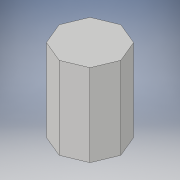
# Autodesk Inventor part: pin_4mm
Saved by Autodesk Inventor 2019 (Build 230136000, 136)
## iProperties
Created: 2019-05-07
Part Number: pin_4mm
Material: Generic
Document SubType Name: Modeling
Designer: assman
Density: 1 g/cm^3
Appearance: Default
Author: assman
Autodesk Inventor part; units mm, degrees
ref_plane "YZ Plane" through (0, 0, 0) normal (1, 0, 0) x (0, 1, 0)
ref_plane "XZ Plane" through (0, 0, 0) normal (0, 1, 0) x (-1, 0, 0)
ref_plane "XY Plane" through (0, 0, 0) normal (0, 0, 1) x (1, 0, 0)
sketch "Sketch1" plane through (0, 0, 0) normal (0, 1, 0) x (-1, 0, 0)
  circle A0 centre (0, 0) radius 1.5 construction
  line L0 (1.5, 0) -> (1.0607, -1.0607)
  line L1 (1.0607, -1.0607) -> (0, -1.5)
  line L2 (0, -1.5) -> (-1.0607, -1.0607)
  line L3 (-1.0607, -1.0607) -> (-1.5, 0)
  line L4 (-1.5, 0) -> (-1.0607, 1.0607)
  line L5 (-1.0607, 1.0607) -> (0, 1.5)
  line L6 (0, 1.5) -> (1.0607, 1.0607)
  line L7 (1.0607, 1.0607) -> (1.5, 0)
  dimension "d0" = 3
  constraints: 16 end point, 2 coincident, 1 horizontal alignment, 19 other
extrude "Extrusion1" add sketch "Sketch1" along normal blind 4
body "Solid1"
